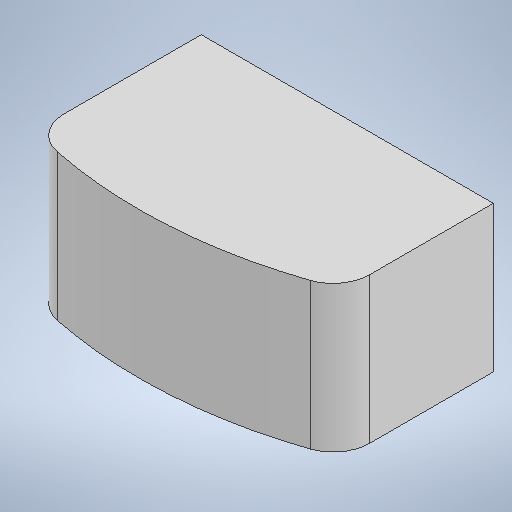
# Autodesk Inventor part: Body01
Saved by Autodesk Inventor 2025 (Build 290162000, 162)
## iProperties
Created: 2024-12-10
Part Number: Body01
Material: Generic
Document SubType Name: Modeling
Designer: naka6
Density: 1 g/cm^3
Appearance: Default
Author: naka6
Autodesk Inventor part; units mm, degrees
ref_plane "YZ Plane" through (0, 0, 0) normal (1, 0, 0) x (0, 1, 0)
ref_plane "XZ Plane" through (0, 0, 0) normal (0, 1, 0) x (-1, 0, 0)
ref_plane "XY Plane" through (0, 0, 0) normal (0, 0, 1) x (1, 0, 0)
sketch "スケッチ1" plane through (0, 0, 0) normal (0, 1, 0) x (-1, 0, 0)
  line L0 (-40, 25) -> (40, 25)
  line L1 (40, 25) -> (40, -25)
  line L2 (40, -25) -> (-40, -25)
  line L3 (-40, -25) -> (-40, 25)
  line L4 (-40, 25) -> (40, -25) construction
  line L5 (40, 25) -> (-40, -25) construction
  circle A0 centre (7, -100) radius 125
  line L6 (40, -15) -> (30, -25)
  point P0 (0, 0)
  point P1 (40, 20.5653)
  point P2 (-40, 15.8275)
  dimension "d0" = 80
  dimension "d1" = 50
  dimension "d2" = 7
  dimension "d3" = 250
  dimension "d6" = 10
  dimension "d7" = 10
  constraints: 14 end point, 2 midpoint, 2 parallel, 2 point on line, 1 centre point, 1 horizontal, 1 perpendicular, 1 tangent
  measures "d0" distance of L0.start L0.end
  measures "d1" distance of L2.end L0.start
  measures "d2" horizontal distance of A0.centre point (0, 0)
  measures "d3" diameter of A0
  measures "d6" distance of L1.end L6.end
  measures "d7" distance of L1.end L6.start
extrude "押し出し1" add sketch "スケッチ1" along normal blind 40 contours A0 L1 L6 L2 L3 | L1 L2 L6
fillet "フィレット1" radius 10 1 edges at (-40, 20, 20.5653)
fillet "フィレット1" radius 10 1 edges at (40, 20, 15.8275)
